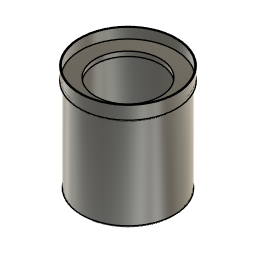
lamp_shade v2 (Autodesk Fusion 360 design; units mm, degrees)
Autodesk Fusion 360 part; units mm, degrees
sketch "Sketch1" plane through (0, 0, 0) normal (0, 0, 1) x (1, 0, 0)
  circle A0 centre (0, 0) radius 50
  dimension "d1" = 100
  constraint coincident A0.centre origin
  measures "d1" diameter of A0
extrude "Extrude1" add sketch "Sketch1" along normal blind 100 thin wall 1 inside
sketch "Sketch2" plane through (0, 0, 0) normal (0, 0, -1) x (1, 0, 0)
  circle A0 centre (0, 0) radius 49
  circle A1 centre (0, 0) radius 50
  circle A2 centre (0, 0) radius 50
  constraint coincident A0.centre A1.centre
extrude "Extrude2" add sketch "Sketch2" against normal blind 1 contours A0
fillet "Fillet1" radius 2 1 edges at (-45.684, 17.7192, 1)
fillet "Fillet2" radius 2 1 edges at (-46.6164, -18.0808, 0)
sketch "Sketch3" plane through (0, 0, 100) normal (0, 0, 1) x (-1, 0, 0)
  circle A0 centre (0, 0) radius 49
  circle A1 centre (0, 0) radius 50
  circle A2 centre (0, 0) radius 52
  circle A3 centre (0, 0) radius 35
  dimension "d11" = 104
  dimension "d12" = 70
  constraint coincident A0.centre A1.centre
  measures "d11" diameter of A2
  measures "d12" diameter of A3
extrude "Extrude3" add sketch "Sketch3" along normal blind 5 contours A0 | A1 | A2
sketch "Sketch4" plane through (0, 0, 105) normal (0, 0, 1) x (-1, 0, 0)
  circle A0 centre (0, 0) radius 35
  circle A1 centre (0, 0) radius 52
  circle A2 centre (0, 0) radius 52
  constraint coincident A0.centre A1.centre
extrude "Extrude4" add sketch "Sketch4" along normal blind 11 thin wall 1 inside contours A0 | A1 A2
fillet "Fillet3" radius 2 1 edges at (48.481, 18.804, 100)
